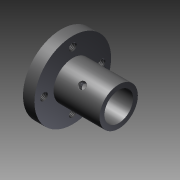
# Autodesk Inventor part: STHRBT15_b
Saved by Autodesk Inventor 2016 (Build 200138000, 138)
## iProperties
Category: PARTsolutions
Company: MISUMI
Created: 2016-06-25
Part Number: STHRBT15_b
Catalog Web Link: www.cadenas.de
Description: STHRBT, STHRT,  SSTHRT_b-Shaft Supports - Bracket Shaped - Standard Tapped Mounting Hole Type - Round Flange
Vendor: MISUMI
Document SubType Name: Modeling
Designer: psAdmin
Manufacturer: MISUMI
Mass: 76.2513 g
Surface Area: 60.1158 cm^2
Volume: 9.53142 cm^3
Density: 8 g/cm^3
Material: ステンレス鋼
Appearance: 半つや出し
PSOL_IDENT_0: {$CADENAS_DATA\23d-libs\misumi\metric\02_shaft_supports\ssthrt\ssthrt_body.prj},188 {VTYP=3D},{NB=ST
PSOL_IDENT_1: HRBT15_b},{LINA=STHRBT15},{NN=STHRBT, STHRT,  SSTHRT_b},{DATE=26.05.2016 07:04:25},{GEOMDATE=21.05.2
PSOL_IDENT_2: 015 00:56:56},{VERSION=},{LINEID=90},{LINESUBID=-1},{WBVAR=MAT,ST,ALT}  {NB=STHRBT15_b},{LINA=STHRBT
PSOL_IDENT_3: 15},{KT=DUMMY},{PN=STHRBT15},{TS=2},{TSALG= '1', 'Drilled Mounting Hole', '2', 'Tapped Mounting Hole'
PSOL_IDENT_4: },{TYPE=STHRBT},{MAT=1018},{MATA= '1018', 'SS400 Equivalent', '304', 'SUS304' },{MALG='M4'},{ST=BO}
PSOL_IDENT_5: ,{ST0= 'BO', 'Black Oxide', 'ENP', 'Electroless Nickel Plating' },{D=15},{THMD11='M4'},{THMD13='M4'}
PSOL_IDENT_6: ,{THMD12='M4'},{DTOL=+0.018/0},{DX=15},{N=2.5},{L=30},{D1=20},{H=40},{T=6.0},{LL=18},{M=M4},{THMD=4}
PSOL_IDENT_7: ,{THMD1=M4},{THMD2=M4},{P=30},{K=32},{W=24},{P1=30},{F=0},{DD1=4.5},{DD11=4.5},{DD12=4.5},{M1=M4},{M
PSOL_IDENT_8: 11=4},{ALT=},{ALTPN=},{BM=4},{BL=3}
NN: STHRBT, STHRT,  SSTHRT_b
NT: Shaft Supports - Bracket Shaped - Standard Tapped Mounting Hole Type - Round Flange
NB: STHRBT15_b
NBSYN: $PN._b
LINA: STHRBT15
PN: STHRBT15
MAT: SS400 Equivalent
ST: Black Oxide
D: 15
DTOL: +0.018/0
N: 2.5
L: 30
D1: 20
H: 40
T: 6.0
LL: 18
M: M4
P: 30
M1: M4
ALT: w/o MB (Hex Socket Set Screw Included)
SUPPLIER: MISUMI
ARTICLENO: STHRBT15_b
BOMINFO: STHRBT15
CREATOR: CADENAS GmbH
Title: STHRBT15
Author: Cadenas PARTsolutions
Comments: Shaft Supports - Bracket Shaped - Standard Tapped Mounting Hole Type - Round Flange
Autodesk Inventor part; units mm, degrees
ref_plane "YZ Plane" through (0, 0, 0) normal (1, 0, 0) x (0, 1, 0)
ref_plane "XZ Plane" through (0, 0, 0) normal (0, 1, 0) x (-1, 0, 0)
ref_plane "XY Plane" through (0, 0, 0) normal (0, 0, 1) x (1, 0, 0)
sketch "Sketch_1" plane through (0, 0, 0) normal (0, 0, 1) x (1, 0, 0)
  line L0 (30, 0) -> (0, 0)
  line L1 (0, 20) -> (0, 7.5)
  line L2 (0, 7.5) -> (30, 7.5)
  line L3 (30, 7.5) -> (30, 10)
  line L4 (30, 10) -> (6, 10)
  line L5 (6, 10) -> (6, 20)
  line L6 (6, 20) -> (0, 20)
  constraints: 14 end point
revolve "Revolution1" add sketch "Sketch_1" angle 360 about axis through (30, 0, 0) along (1, 0, 0)
sketch "Sketch_3" plane through (0, 0, 0) normal (0, -0.7071, 0.7071) x (1, 0, 0)
  line L0 (18, 7) -> (18, 10)
  line L1 (18, 10) -> (20, 10)
  line L2 (20, 10) -> (19.621, 9.621)
  line L3 (19.621, 9.621) -> (19.621, 7)
  line L4 (19.621, 7) -> (18, 7)
  line L5 (18, 7) -> (18, 10)
  constraints: 12 end point
revolve "Revolution2" cut sketch "Sketch_3" angle 360 about axis through (18, 4.9497, 4.9497) along (0, -0.7071, -0.7071)
thread "Thread1" size "M4x0.7" class "6H" standard "ISO Metric profile" length 2.621
sketch "Sketch_2" plane through (0, 0, 0) normal (0, -0.7071, -0.7071) x (1, 0, 0)
  line L0 (18, 7) -> (18, 10)
  line L1 (18, 10) -> (20, 10)
  line L2 (20, 10) -> (19.621, 9.621)
  line L3 (19.621, 9.621) -> (19.621, 7)
  line L4 (19.621, 7) -> (18, 7)
  line L5 (18, 7) -> (18, 10)
  constraints: 12 end point
revolve "Revolution3" cut sketch "Sketch_2" angle 360 about axis through (18, -4.9497, 4.9497) along (0, 0.7071, -0.7071)
thread "Thread2" size "M4x0.7" class "6H" standard "ISO Metric profile" length 2.621
sketch "Sketch_4" plane through (0, 0, 0) normal (0, 0, 1) x (1, 0, 0)
  line L0 (6, 15) -> (0, 15)
  line L1 (0, 15) -> (0, 17)
  line L2 (0, 17) -> (0.379, 16.621)
  line L3 (0.379, 16.621) -> (5.621, 16.621)
  line L4 (5.621, 16.621) -> (6, 17)
  line L5 (6, 17) -> (6, 15)
  line L6 (6, 15) -> (0, 15)
  constraints: 14 end point
revolve "Revolution4" cut sketch "Sketch_4" angle 360 about axis through (6, 15, 0) along (1, 0, 0)
thread "Thread3" size "M4x0.7" class "6H" standard "ISO Metric profile" full length
sketch "Sketch_9" plane through (0, 0, 0) normal (0, -1, 0) x (1, 0, 0)
  line L0 (0, -15) -> (6, -15)
  line L1 (6, -15) -> (6, -17)
  line L2 (6, -17) -> (5.621, -16.621)
  line L3 (5.621, -16.621) -> (0.379, -16.621)
  line L4 (0.379, -16.621) -> (0, -17)
  line L5 (0, -17) -> (0, -15)
  line L6 (0, -15) -> (6, -15)
  constraints: 14 end point
revolve "Revolution5" cut sketch "Sketch_9" angle 360 about axis through (0, 0, -15) along (-1, 0, 0)
thread "Thread4" size "M4x0.7" class "6H" standard "ISO Metric profile" full length
sketch "Sketch_10" plane through (0, 0, 0) normal (0, 0, 1) x (1, 0, 0)
  line L0 (0, -15) -> (6, -15)
  line L1 (6, -15) -> (6, -17)
  line L2 (6, -17) -> (5.621, -16.621)
  line L3 (5.621, -16.621) -> (0.379, -16.621)
  line L4 (0.379, -16.621) -> (0, -17)
  line L5 (0, -17) -> (0, -15)
  line L6 (0, -15) -> (6, -15)
  constraints: 14 end point
revolve "Revolution6" cut sketch "Sketch_10" angle 360 about axis through (0, -15, 0) along (-1, 0, 0)
thread "Thread5" size "M4x0.7" class "6H" standard "ISO Metric profile" full length
sketch "Sketch_11" plane through (0, 0, 0) normal (0, -1, 0) x (1, 0, 0)
  line L0 (6, 15) -> (0, 15)
  line L1 (0, 15) -> (0, 17)
  line L2 (0, 17) -> (0.379, 16.621)
  line L3 (0.379, 16.621) -> (5.621, 16.621)
  line L4 (5.621, 16.621) -> (6, 17)
  line L5 (6, 17) -> (6, 15)
  line L6 (6, 15) -> (0, 15)
  constraints: 14 end point
revolve "Revolution7" cut sketch "Sketch_11" angle 360 about axis through (6, 0, 15) along (1, 0, 0)
thread "Thread6" size "M4x0.7" class "6H" standard "ISO Metric profile" full length
body "Solid1"
